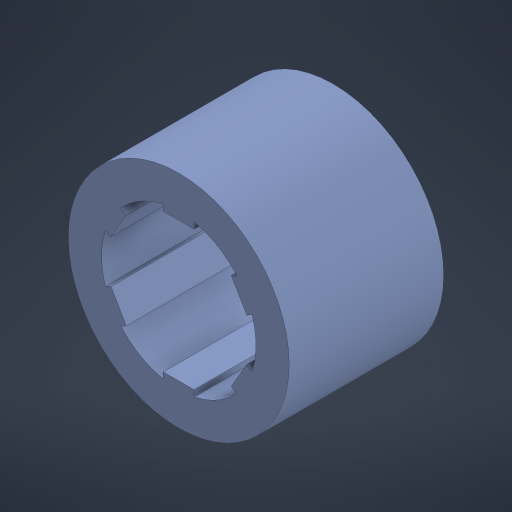
# Autodesk Inventor part: opona
Saved by Autodesk Inventor 2023.4 (Build 274418000, 418)
## iProperties
Created: 2025-11-07
Part Number: opona
Material: Rubber, Silicone
Document SubType Name: Modeling
Designer: borsu
Density: 1.25 g/cm^3
Appearance: Rubber - Blue
Author: borsu
Autodesk Inventor part; units mm, degrees
ref_plane "YZ Plane" through (0, 0, 0) normal (1, 0, 0) x (0, 1, 0)
ref_plane "XZ Plane" through (0, 0, 0) normal (0, 1, 0) x (-1, 0, 0)
ref_plane "XY Plane" through (0, 0, 0) normal (0, 0, 1) x (1, 0, 0)
sketch "Sketch1" plane through (0, 0, 0) normal (0, 0, 1) x (1, 0, 0)
  line L0 (0, -20.02) -> (0, 20.02) projected
  line L1 (-20.02, 0) -> (20.02, 0) projected
  circle A0 centre (0, 0) radius 10
  circle A1 centre (0, 0) radius 14.3
  line L2 (-2, 9) -> (2, 9)
  line L3 (2, 9) -> (2, 11)
  line L4 (2, 11) -> (-2, 11)
  line L5 (-2, 11) -> (-2, 9)
  line L6 (-2, 9) -> (2, 11) construction
  line L7 (2, 9) -> (-2, 11) construction
  line L8 (6.7942, 6.2321) -> (8.7942, 2.7679)
  line L9 (8.7942, 2.7679) -> (10.5263, 3.7679)
  line L10 (10.5263, 3.7679) -> (8.5263, 7.2321)
  line L11 (8.5263, 7.2321) -> (6.7942, 6.2321)
  line L12 (6.7942, 6.2321) -> (10.5263, 3.7679) construction
  line L13 (8.7942, 2.7679) -> (8.5263, 7.2321) construction
  line L14 (8.7942, -2.7679) -> (6.7942, -6.2321)
  line L15 (6.7942, -6.2321) -> (8.5263, -7.2321)
  line L16 (8.5263, -7.2321) -> (10.5263, -3.7679)
  line L17 (10.5263, -3.7679) -> (8.7942, -2.7679)
  line L18 (8.7942, -2.7679) -> (8.5263, -7.2321) construction
  line L19 (6.7942, -6.2321) -> (10.5263, -3.7679) construction
  line L20 (2, -9) -> (-2, -9)
  line L21 (-2, -9) -> (-2, -11)
  line L22 (-2, -11) -> (2, -11)
  line L23 (2, -11) -> (2, -9)
  line L24 (2, -9) -> (-2, -11) construction
  line L25 (-2, -9) -> (2, -11) construction
  line L26 (-6.7942, -6.2321) -> (-8.7942, -2.7679)
  line L27 (-8.7942, -2.7679) -> (-10.5263, -3.7679)
  line L28 (-10.5263, -3.7679) -> (-8.5263, -7.2321)
  line L29 (-8.5263, -7.2321) -> (-6.7942, -6.2321)
  line L30 (-6.7942, -6.2321) -> (-10.5263, -3.7679) construction
  line L31 (-8.7942, -2.7679) -> (-8.5263, -7.2321) construction
  line L32 (-8.7942, 2.7679) -> (-6.7942, 6.2321)
  line L33 (-6.7942, 6.2321) -> (-8.5263, 7.2321)
  line L34 (-8.5263, 7.2321) -> (-10.5263, 3.7679)
  line L35 (-10.5263, 3.7679) -> (-8.7942, 2.7679)
  line L36 (-8.7942, 2.7679) -> (-8.5263, 7.2321) construction
  line L37 (-6.7942, 6.2321) -> (-10.5263, 3.7679) construction
  point P0 (0, 10)
  point P1 (8.6603, 5)
  point P2 (8.6603, -5)
  point P3 (0, -10)
  point P4 (-8.6603, -5)
  point P5 (-8.6603, 5)
  point P6 (-7.4853, 6.631)
  point P7 (-2, 9.798)
  point P8 (2, 9.798)
  point P9 (7.4853, 6.631)
  point P10 (9.4853, 3.1669)
  point P11 (9.4853, -3.1669)
  point P12 (7.4853, -6.631)
  point P13 (2, -9.798)
  point P14 (-2, -9.798)
  point P15 (-7.4853, -6.631)
  point P16 (-9.4853, -3.1669)
  point P17 (-9.4853, 3.1669)
  dimension "d0" = 20
  dimension "d1" = 28.6
  dimension "d2" = 4
  dimension "d3" = 2
  dimension "d6" = 360
  constraints: 72 end point, 4 coincident, 2 midpoint, 2 parallel, 1 centre point, 1 horizontal, 1 perpendicular, 1 point on line, 74 other
  measures "d1" diameter of A1
  measures "d2" distance of L3.end L4.end
  measures "d3" distance of L2.end L3.end
extrude "Extrusion1" add sketch "Sketch1" along normal blind 20 contours A1 L1 A0 L27 L28 L29 L21 L22 L0 | L0 L22 L23 A0 L15 L16 L17 L1 A1 | L22 L21 A0 L0 | L0 A0 L23 L22 | A1 L0 L4 L5 A0 L33 L34 L35 L1 | L1 A0 L9 L10 L11 L3 L4 L0 A1 | A0 L21 L20 L0 | L0 L20 L23 A0 | L35 L34 L33 A0 | A0 L33 L32 L35 | L27 L26 L29 A0 | A0 L29 L28 L27 | L4 L3 A0 L0 | L0 A0 L5 L4 | L9 L8 L11 A0 | A0 L11 L10 L9 | L17 L16 L15 A0 | A0 L15 L14 L17 | L2 L5 A0 L0 | L0 A0 L3 L2
body "Solid1"
